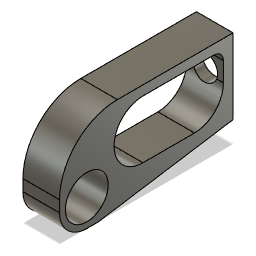
Connector 2 v1 (Autodesk Fusion 360 design; units mm, degrees)
Autodesk Fusion 360 part; units mm, degrees
sketch "Sketch1" plane through (0, 0, 0) normal (0, 1, 0) x (1, 0, 0)
  line L0 (0, 0) -> (19, 0)
  line L1 (19, 0) -> (19, 90)
  line L2 (19, 90) -> (0, 90)
  line L3 (0, 90) -> (0, 0)
  dimension "d1" = 19
  dimension "d2" = 90
  constraint horizontal L0
  constraint vertical L1
  constraint horizontal L2
  constraint vertical L3
  constraint coincident L0.start L3.end
  measures "d1" distance of L0.start L0.end
  measures "d2" distance of L0.start L2.end
extrude "Extrude1" add sketch "Sketch1" along normal blind 50
sketch "Sketch2" plane through (19, 0, 0) normal (1, 0, 0) x (0, 0, -1)
  line L0 (0, 0) -> (90, 0)
  line L1 (90, 0) -> (90, 50)
  line L2 (90, 50) -> (0, 50)
  line L3 (0, 50) -> (0, 0)
  circle A0 centre (14.125, 14.125) radius 11.125
  line L4 (28.25, 45) -> (85, 45)
  line L5 (85, 45) -> (85, 15)
  line L6 (85, 15) -> (28.25, 15)
  line L7 (28.25, 15) -> (28.25, 45)
  circle A1 centre (14.125, 14.125) radius 14.125
  dimension "d5" = 22.25
  dimension "d7" = 5
  dimension "d8" = 15
  dimension "d9" = 5
  dimension "d10" = 30
  dimension "d24" = 3
  constraint horizontal L4
  constraint vertical L5
  constraint horizontal L6
  constraint vertical L7
  constraint tangent L3 A1
  constraint tangent L0 A1
  constraint tangent L7 A1
  measures "d5" diameter of A0
  measures "d7" distance of L2 L4
  measures "d8" distance of L0 L6
  measures "d9" distance of L1 L5
  measures "d10" distance of L4 L6
extrude "Extrude2" cut sketch "Sketch2" against normal up to surface (19 mm away) contours L0 L3 A1 | A0 | L4 L5 L6 L7
fillet "Fillet1" radius 30 1 edges at (9.5, 50, 0)
sketch "Sketch3" plane through (0, 0, -90) normal (0, 0, -1) x (-1, 0, 0)
  line L0 (-19, 0) -> (0, 0)
  line L1 (0, 0) -> (0, 50)
  line L2 (0, 50) -> (-19, 50)
  line L3 (-19, 50) -> (-19, 0)
  circle A0 centre (-9.5, 32.5) radius 6.5
  line L4 (-9.5, 50) -> (-9.5, 0) construction
  line L5 (-19, 32.5) -> (0, 32.5) construction
  dimension "d17" = 13
  dimension "d29" = 17.5
  constraint midpoint L2 L4.start
  constraint midpoint L0 L4.end
  constraint coincident A0.centre L4
  constraint coincident A0.centre L5
  constraint horizontal L5
  constraint coincident L3 L5.start
  constraint coincident L1 L5.end
  measures "d17" diameter of A0
  measures "d29" distance of L2 L5
extrude "Extrude3" cut sketch "Sketch3" against normal up to surface (5 mm away) contours A0
fillet "Fillet2" radius 15 1 edges at (9.5, 15, -85)
fillet "Fillet2" radius 5 1 edges at (9.5, 45, -85)
fillet "Fillet3" radius 15 2 edges at (9.5, 45, -28.25) (9.5, 15, -28.25)
chamfer "Chamfer1" distance 11 distance2 70 1 edges at (9.5, 0, -90) measured on face at (9.6619, 8.6727, -90)
equation "d6 = d5"
